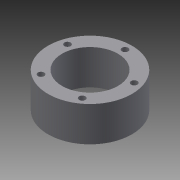
# Autodesk Inventor part: drive wheel sprocket spacer
Saved by Autodesk Inventor 2014 (Build 180170000, 170)
## iProperties
Created: 2015-09-16
Part Number: drive wheel sprocket spacer
Material: Generic
Document SubType Name: Modeling
Designer: zimirken
Density: 1 g/cm^3
Appearance: Default
Author: zimirken
Autodesk Inventor part; units mm, degrees
ref_plane "YZ Plane" through (0, 0, 0) normal (1, 0, 0) x (0, 1, 0)
ref_plane "XZ Plane" through (0, 0, 0) normal (0, 1, 0) x (-1, 0, 0)
ref_plane "XY Plane" through (0, 0, 0) normal (0, 0, 1) x (1, 0, 0)
sketch "Sketch1" plane through (0, 0, 0) normal (0, 0, 1) x (1, 0, 0)
  line L0 (0, 50.2073) -> (47.75, 15.5149) construction
  line L1 (47.75, 15.5149) -> (29.5111, -40.6186) construction
  line L2 (29.5111, -40.6186) -> (-29.5111, -40.6186) construction
  line L3 (-29.5111, -40.6186) -> (-47.75, 15.5149) construction
  line L4 (-47.75, 15.5149) -> (0, 50.2073) construction
  circle A0 centre (0, 50.2073) radius 4.5
  circle A1 centre (47.75, 15.5149) radius 4.5
  circle A2 centre (29.5111, -40.6186) radius 4.5
  circle A3 centre (-29.5111, -40.6186) radius 4.5
  circle A4 centre (-47.75, 15.5149) radius 4.5
  circle A5 centre (0, 0) radius 40
  circle A6 centre (0, 0) radius 60
  dimension "d0" = 95.5
  dimension "d1" = 9
  dimension "d2" = 80
  dimension "d3" = 120
  constraints: 10 end point, 8 coincident, 7 centre point, 4 equal radius, 1 horizontal, 11 other
  measures "d0" distance of L0.end L3.end
  measures "d1" diameter of A0
  measures "d2" diameter of A5
  measures "d3" diameter of A6
extrude "Extrusion1" add sketch "Sketch1" along normal blind 50
body "Solid1"
